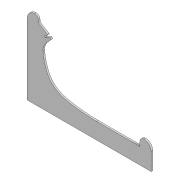
# Autodesk Inventor part: steep-rail
Saved by Autodesk Inventor 2020 (Build 240168000, 168)
## iProperties
Created: 2021-06-11
Part Number: steep-rail
Material: Generic
Document SubType Name: Modeling
Designer: Aidan Lee
Density: 1 g/cm^3
Appearance: Default
Author: Aidan Lee
Autodesk Inventor part; units mm, degrees
ref_plane "YZ Plane" through (0, 0, 0) normal (1, 0, 0) x (0, 1, 0)
ref_plane "XZ Plane" through (0, 0, 0) normal (0, 1, 0) x (-1, 0, 0)
ref_plane "XY Plane" through (0, 0, 0) normal (0, 0, 1) x (1, 0, 0)
sketch "Sketch3" plane through (0, 0, 0) normal (0, 0, 1) x (1, 0, 0)
  circle A0 centre (368.0481, 50) radius 50 construction
  line L0 (368.0481, 0) -> (514.9541, 0) construction
  line L1 (368.0481, 50) -> (514.9541, 50) construction
  line L2 (368.0481, 100) -> (514.9541, 100) construction
  line L3 (368.0481, 50) -> (343.0481, 6.6987) construction
  line L4 (368.0481, 50) -> (324.7469, 25) construction
  line L5 (368.0481, 50) -> (324.7469, 75) construction
  line L6 (343.0481, 93.3013) -> (368.0481, 50) construction
  line L7 (393.0481, 93.3013) -> (368.0481, 50) construction
  line L8 (411.3494, 75) -> (368.0481, 50) construction
  line L9 (411.3494, 25) -> (368.0481, 50) construction
  line L10 (393.0481, 6.6987) -> (368.0481, 50) construction
  line L11 (368.0481, 0) -> (368.0481, 100) construction
  line L12 (418.0481, 50) -> (368.0481, 50) construction
  line L13 (341.8682, 0) -> (341.8682, 100) construction
  line L14 (315.6883, 0) -> (315.6883, 100) construction
  line L15 (289.5083, 0) -> (289.5083, 100) construction
  line L16 (263.3284, 0) -> (263.3284, 100) construction
  line L17 (237.1485, 0) -> (237.1485, 100) construction
  line L18 (210.9685, 0) -> (210.9685, 100) construction
  line L19 (184.7886, 0) -> (184.7886, 100) construction
  line L20 (158.6086, 0) -> (158.6086, 100) construction
  circle A1 centre (315.6883, 50) radius 50 construction
  circle A2 centre (341.8682, 50) radius 50 construction
  circle A3 centre (289.5083, 50) radius 50 construction
  circle A4 centre (263.3284, 50) radius 50 construction
  circle A5 centre (237.1485, 50) radius 50 construction
  circle A6 centre (210.9685, 50) radius 50 construction
  line L21 (393.0481, 6.6987) -> (514.9541, 6.6987) construction
  line L22 (411.3494, 25) -> (514.9541, 25) construction
  line L23 (411.3494, 75) -> (514.9541, 75) construction
  line L24 (411.3494, 75) -> (514.9541, 75) construction
  line L25 (393.0481, 93.3013) -> (514.9541, 93.3013) construction
  line L26 (358.9895, 75) -> (339.5083, 50) construction
  line L27 (339.5083, 50) -> (306.6297, 25) construction
  line L28 (306.6297, 25) -> (262.1485, 6.6987) construction
  line L29 (262.1485, 6.6987) -> (210.9685, 0) construction
  line L30 (105.4843, -12.0642) -> (105.4843, 125.3083) construction
  line L31 (25.75, 0) -> (25.75, 23)
  line L32 (45.75, 17) -> (45.75, -21.2379)
  arc A7 (32.75, 30) -> (25.75, 23) centre (32.75, 23) ccw
  arc A8 (45.75, 17) -> (32.75, 30) centre (32.75, 17) ccw
  line L33 (32.75, 17) -> (45.75, 17) construction
  line L34 (32.75, 17) -> (32.75, 30) construction
  arc A9 (0, 0) -> (8.875, -12.2379) centre (12.875, 0) ccw
  arc A10 (16.875, -12.2379) -> (25.75, 0) centre (12.875, 0) ccw
  line L35 (45.75, -21.2379) -> (16.875, -21.2379)
  line L36 (8.875, -21.2379) -> (-177.0796, -21.2379)
  circle A11 centre (-144.2046, 110.3653) radius 12.875 construction
  line L37 (8.875, -21.2379) -> (8.875, -12.2379)
  line L38 (16.875, -21.2379) -> (16.875, -12.2379)
  line L39 (411.3494, 75) -> (158.6086, 75) construction
  line L40 (368.0481, 100) -> (158.6086, 100) construction
  line L41 (418.0481, 50) -> (158.6086, 50) construction
  line L42 (411.3494, 25) -> (158.6086, 25) construction
  line L43 (393.0481, 6.6987) -> (158.6086, 6.6987) construction
  line L44 (393.0481, 93.3013) -> (158.6086, 93.3013) construction
  line L45 (358.9895, 75) -> (366.8682, 93.3013) construction
  line L46 (366.8682, 93.3013) -> (368.0481, 100) construction
  spline S0 degree 4 poles (-157.0796, 100) (-157.0796, 88.9946) (-147.011, 72.6811) (-131.8577, 48.7932) (-88.4777, 17.6268) (-50.0176, 3.937) (-18.8717, 0) (0, 0) knots 0 0 0 0 0 0.264547 0.457223 0.66608 1 1 1 1 1
  line L47 (-157.0796, 100) -> (-157.0796, 81.2146) construction
  line L48 (0, 0) -> (-42.8818, 0) construction
  line L49 (-157.0796, 100) -> (-157.0796, 113)
  line L50 (-144.2046, 110.3653) -> (-157.0796, 110.3653) construction
  line L51 (-147.6984, 94.0277) -> (-120.1158, 108.3975) construction
  line L52 (-157.0796, 100) -> (0, 0) construction
  circle A12 centre (-147.2046, 105.4197) radius 9.875 construction
  line L53 (-147.2046, 105.4197) -> (-157.0796, 105.4197) construction
  line L54 (-146.1623, 94.828) -> (-144.7762, 92.1674) construction
  line L55 (-144.7762, 92.1674) -> (-142.2689, 93.4736) construction
  line L56 (-177.0796, 107) -> (-177.0796, -21.2379)
  arc A13 (-157.0796, 113) -> (-164.0796, 120) centre (-164.0796, 113) ccw
  line L57 (-164.0796, 113) -> (-164.0796, 120) construction
  line L58 (-164.0796, 113) -> (-157.0796, 113) construction
  arc A14 (-164.0796, 120) -> (-177.0796, 107) centre (-164.0796, 107) ccw
  line L59 (-164.0796, 107) -> (-177.0796, 107) construction
  line L60 (-164.0796, 107) -> (-164.0796, 120) construction
  line L61 (-457.0796, 100) -> (-300, 0)
  line L62 (-757.0796, 100) -> (-757.0796, 76.4376)
  line L63 (-600, 0) -> (-652.3765, 0)
  spline S1 degree 4 poles (-757.0796, 76.4376) (-757.0796, 65.0585) (-753.7776, 47.1407) (-745.4013, 7.8331) (-693.0053, 2.4317) (-668.8587, 0) (-652.3765, 0) knots 0 0 0 0 0 0.348765 0.598765 1 1 1 1 1
  line L64 (-477.0796, 107) -> (-477.0796, -21.2379)
  arc A15 (-464.0796, 120) -> (-477.0796, 107) centre (-464.0796, 107) ccw
  arc A16 (-457.0796, 113) -> (-464.0796, 120) centre (-464.0796, 113) ccw
  line L65 (-457.0796, 100) -> (-457.0796, 113)
  circle A17 centre (-447.2046, 105.4197) radius 9.875 construction
  circle A18 centre (-444.2046, 110.3653) radius 12.875 construction
  line L66 (-457.0796, 100) -> (-300, 0) construction
  line L67 (-447.6984, 94.0277) -> (-420.1158, 108.3975) construction
  line L68 (-444.7762, 92.1674) -> (-442.2689, 93.4736) construction
  line L69 (-446.1623, 94.828) -> (-444.7762, 92.1674) construction
  line L70 (-291.125, -21.2379) -> (-477.0796, -21.2379)
  arc A19 (-300, 0) -> (-291.125, -12.2379) centre (-287.125, 0) ccw
  line L71 (-291.125, -21.2379) -> (-291.125, -12.2379)
  line L72 (-283.125, -21.2379) -> (-283.125, -12.2379)
  arc A20 (-283.125, -12.2379) -> (-274.25, 0) centre (-287.125, 0) ccw
  line L73 (-254.25, -21.2379) -> (-283.125, -21.2379)
  line L74 (-254.25, 17) -> (-254.25, -21.2379)
  line L75 (-274.25, 0) -> (-274.25, 23)
  arc A21 (-267.25, 30) -> (-274.25, 23) centre (-267.25, 23) ccw
  arc A22 (-254.25, 17) -> (-267.25, 30) centre (-267.25, 17) ccw
  line L76 (-777.0796, 107) -> (-777.0796, -21.2379)
  arc A23 (-764.0796, 120) -> (-777.0796, 107) centre (-764.0796, 107) ccw
  arc A24 (-757.0796, 113) -> (-764.0796, 120) centre (-764.0796, 113) ccw
  line L77 (-757.0796, 100) -> (-757.0796, 113)
  circle A25 centre (-747.2046, 105.4197) radius 9.875 construction
  circle A26 centre (-744.2046, 110.3653) radius 12.875 construction
  line L78 (-757.0796, 100) -> (-600, 0) construction
  line L79 (-747.6984, 94.0277) -> (-720.1158, 108.3975) construction
  line L80 (-744.7762, 92.1674) -> (-742.2689, 93.4736) construction
  line L81 (-746.1623, 94.828) -> (-744.7762, 92.1674) construction
  line L82 (-591.125, -21.2379) -> (-777.0796, -21.2379)
  arc A27 (-600, 0) -> (-591.125, -12.2379) centre (-587.125, 0) ccw
  line L83 (-591.125, -21.2379) -> (-591.125, -12.2379)
  line L84 (-583.125, -21.2379) -> (-583.125, -12.2379)
  arc A28 (-583.125, -12.2379) -> (-574.25, 0) centre (-587.125, 0) ccw
  line L85 (-554.25, -21.2379) -> (-583.125, -21.2379)
  line L86 (-554.25, 17) -> (-554.25, -21.2379)
  line L87 (-574.25, 0) -> (-574.25, 23)
  arc A29 (-567.25, 30) -> (-574.25, 23) centre (-567.25, 23) ccw
  arc A30 (-554.25, 17) -> (-567.25, 30) centre (-567.25, 17) ccw
  line L88 (32.75, -233) -> (45.75, -233) construction
  line L89 (32.75, -233) -> (32.75, -220) construction
  arc A31 (45.75, -233) -> (32.75, -220) centre (32.75, -233) ccw construction
  line L90 (25.75, -250) -> (25.75, -227) construction
  line L91 (45.75, -233) -> (45.75, -271.2379) construction
  arc A32 (16.875, -262.2379) -> (25.75, -250) centre (12.875, -250) ccw construction
  line L92 (45.75, -271.2379) -> (16.875, -271.2379) construction
  arc A33 (0, -250) -> (8.875, -262.2379) centre (12.875, -250) ccw construction
  arc A34 (32.75, -220) -> (25.75, -227) centre (32.75, -227) ccw construction
  line L93 (8.875, -271.2379) -> (-177.0796, -271.2379) construction
  line L94 (-157.0796, -150) -> (0, -250) construction
  spline S2 degree 4 poles (-157.0796, -150) (-157.0796, -161.0054) (-147.011, -177.3189) (-131.8577, -201.2068) (-88.4777, -232.3732) (-50.0176, -246.063) (-18.8717, -250) (0, -250) knots 0 0 0 0 0 0.264547 0.457223 0.66608 1 1 1 1 1 construction
  line L95 (-177.0796, -143) -> (-177.0796, -271.2379)
  line L96 (-146.1623, -155.172) -> (-144.7762, -157.8326) construction
  line L97 (-144.7762, -157.8326) -> (-142.2689, -156.5264) construction
  line L98 (-147.6984, -155.9723) -> (-120.1158, -141.6025) construction
  line L99 (-157.0796, -150) -> (-157.0796, -168.7854) construction
  line L100 (-147.2046, -144.5803) -> (-157.0796, -144.5803) construction
  line L101 (-144.2046, -139.6347) -> (-157.0796, -139.6347) construction
  circle A35 centre (-147.2046, -144.5803) radius 9.875 construction
  line L102 (0, -250) -> (-42.8818, -250) construction
  line L103 (16.875, -271.2379) -> (16.875, -262.2379) construction
  line L104 (8.875, -271.2379) -> (8.875, -262.2379) construction
  circle A36 centre (-144.2046, -139.6347) radius 12.875 construction
  line L105 (-164.0796, -143) -> (-177.0796, -143) construction
  line L106 (-157.0796, -150) -> (-157.0796, -137) construction
  line L107 (-164.0796, -137) -> (-157.0796, -137) construction
  arc A37 (-157.0796, -137) -> (-164.0796, -130) centre (-164.0796, -137) ccw
  line L108 (-164.0796, -137) -> (-164.0796, -130) construction
  line L109 (-164.0796, -143) -> (-164.0796, -130) construction
  arc A38 (-164.0796, -130) -> (-177.0796, -143) centre (-164.0796, -143) ccw
  arc A39 (32.75, -227) -> (25.75, -234) centre (32.75, -234) ccw
  line L110 (32.75, -234) -> (25.75, -234) construction
  line L111 (32.75, -234) -> (32.75, -227) construction
  line L112 (45.75, -271.2379) -> (-177.0796, -271.2379)
  arc A40 (45.75, -240) -> (32.75, -227) centre (32.75, -240) ccw
  line L113 (32.75, -240) -> (45.75, -240) construction
  line L114 (32.75, -240) -> (32.75, -227) construction
  line L115 (45.75, -240) -> (45.75, -271.2379)
  line L116 (0, -242) -> (25.75, -242)
  line L117 (25.75, -234) -> (25.75, -242)
  line L118 (-149.0796, -145.6094) -> (-149.0796, -150)
  line L119 (-149.0796, -145.6094) -> (-157.0796, -140.5164)
  line L120 (-157.0796, -140.5164) -> (-157.0796, -137)
  line L121 (57.9242, -250) -> (-50.1018, -250) construction
  spline S3 degree 4 poles (-149.0796, -150) (-149.0796, -154.1011) (-147.2668, -159.7716) (-135.8793, -178.0796) (-120.229, -197.0865) (-83.3361, -225.9308) (-47.2959, -235.9761) (-18.0598, -242) (0, -242) knots 0 0 0 0 0 0.173174 0.31592 0.488873 0.682943 1 1 1 1 1
  line L122 (-158.9844, -148.7874) -> (-160.5796, -147.7718) construction
  line L123 (-149.0796, -145.6094) -> (2.3304, -242) construction
  line L124 (-149.0796, -145.6094) -> (-139.5059, -151.7042)
  line L125 (-146.1623, -155.172) -> (-139.5059, -151.7042)
  line L126 (-144.7762, -157.8326) -> (-146.1623, -155.172)
  line L127 (-144.7762, -157.8326) -> (-136.5837, -153.5646)
  line L128 (-136.5837, -153.5646) -> (-134.053, -155.1756)
  line L129 (-136.5837, -153.5646) -> (-136.7042, -153.7538) construction
  line L130 (-134.053, -155.1756) -> (-134.1481, -155.3251) construction
  spline S4 degree 4 poles (-134.053, -155.1756) (-136.3893, -157.4676) (-136.0613, -162.1246) (-140.7447, -169.8773) (-137.1035, -175.12) knots 0 0 0 0 0 1 1 1 1 1
  line L131 (-134.053, -155.1756) -> (-131.4385, -154.0999) construction
  line L132 (-254.25, -271.2379) -> (-477.0796, -271.2379)
  line L133 (-477.0796, -143) -> (-477.0796, -271.2379)
  arc A41 (-464.0796, -130) -> (-477.0796, -143) centre (-464.0796, -143) ccw
  arc A42 (-457.0796, -137) -> (-464.0796, -130) centre (-464.0796, -137) ccw
  line L134 (-457.0796, -140.5164) -> (-457.0796, -137)
  line L135 (-449.0796, -145.6094) -> (-457.0796, -140.5164)
  line L136 (-449.0796, -145.6094) -> (-439.5059, -151.7042)
  line L137 (-446.1623, -155.172) -> (-439.5059, -151.7042)
  line L138 (-444.7762, -157.8326) -> (-446.1623, -155.172)
  line L139 (-444.7762, -157.8326) -> (-436.5837, -153.5646)
  line L140 (-436.5837, -153.5646) -> (-434.053, -155.1756)
  line L141 (-449.0796, -145.6094) -> (-297.6696, -242) construction
  line L142 (-300, -242) -> (-274.25, -242)
  line L143 (-274.25, -234) -> (-274.25, -242)
  arc A43 (-267.25, -227) -> (-274.25, -234) centre (-267.25, -234) ccw
  arc A44 (-254.25, -240) -> (-267.25, -227) centre (-267.25, -240) ccw
  line L144 (-254.25, -240) -> (-254.25, -271.2379)
  circle A45 centre (-447.2046, -144.5803) radius 9.875 construction
  line L145 (-457.0796, -150) -> (-300, -250) construction
  circle A46 centre (-444.2046, -139.6347) radius 12.875 construction
  line L146 (-554.25, -271.2379) -> (-777.0796, -271.2379)
  line L147 (-777.0796, -143) -> (-777.0796, -271.2379)
  arc A47 (-764.0796, -130) -> (-777.0796, -143) centre (-764.0796, -143) ccw
  arc A48 (-757.0796, -137) -> (-764.0796, -130) centre (-764.0796, -137) ccw
  line L148 (-757.0796, -140.5164) -> (-757.0796, -137)
  line L149 (-749.0796, -145.6094) -> (-757.0796, -140.5164)
  line L150 (-749.0796, -145.6094) -> (-739.5059, -151.7042)
  line L151 (-746.1623, -155.172) -> (-739.5059, -151.7042)
  line L152 (-744.7762, -157.8326) -> (-746.1623, -155.172)
  line L153 (-744.7762, -157.8326) -> (-736.5837, -153.5646)
  line L154 (-736.5837, -153.5646) -> (-734.053, -155.1756)
  line L155 (-749.0796, -145.6094) -> (-597.6696, -242) construction
  line L156 (-600, -242) -> (-574.25, -242)
  line L157 (-574.25, -234) -> (-574.25, -242)
  arc A49 (-567.25, -227) -> (-574.25, -234) centre (-567.25, -234) ccw
  arc A50 (-554.25, -240) -> (-567.25, -227) centre (-567.25, -240) ccw
  line L158 (-554.25, -240) -> (-554.25, -271.2379)
  circle A51 centre (-747.2046, -144.5803) radius 9.875 construction
  line L159 (-757.0796, -150) -> (-600, -250) construction
  circle A52 centre (-744.2046, -139.6347) radius 12.875 construction
  line L160 (-297.6696, -242) -> (-434.053, -155.1756)
  spline S5 degree 4 poles (-757.0796, -173.5624) (-757.0796, -184.9415) (-753.7776, -202.8593) (-745.4013, -242.1669) (-693.0053, -247.5683) (-668.8587, -250) (-652.3765, -250) knots 0 0 0 0 0 0.348765 0.598765 1 1 1 1 1 construction
  line L161 (-757.0796, -150) -> (-757.0796, -173.5624)
  line L162 (-600, -250) -> (-652.3765, -250) construction
  line L163 (-600, -242) -> (-652.3765, -242)
  spline S6 degree 4 poles (-749.0796, -173.5624) (-749.0796, -183.7991) (-746.0176, -199.7502) (-737.9559, -236.335) (-690.8375, -239.2991) (-667.8077, -242) (-652.3765, -242) knots 0 0 0 0 0 0.346383 0.596383 1 1 1 1 1
  line L164 (-749.0796, -173.5624) -> (-749.0796, -170.035) construction
  spline S7 degree 3 poles (-734.053, -155.1756) (-737.3254, -159.7583) (-749.7015, -168.859) (-748.818, -180.0805) knots 0 0 0 0 1 1 1 1
  point P0 (158.6086, 0)
  point P1 (-148.021, 75)
  point P2 (-128.5398, 50)
  point P3 (-95.6611, 25)
  point P4 (-51.1799, 6.6987)
  point P5 (-155.8997, 93.3013)
  point P6 (-753.2027, 48.1984)
  point P7 (-737.7866, 19.9116)
  point P8 (-697.6619, 3.8098)
  point P9 (-457.0796, 110.3653)
  point P10 (-457.0796, 105.4197)
  point P11 (-757.0796, 110.3653)
  point P12 (-757.0796, 105.4197)
  point P13 (-51.1799, -243.3013)
  point P14 (-95.6611, -225)
  point P15 (-148.021, -175)
  point P16 (-128.5398, -200)
  point P17 (-155.8997, -156.6987)
  point P18 (-157.0796, -141.4334)
  point P19 (-153.0796, -143.0629)
  point P20 (-152.1421, -144.5803)
  point P21 (3.9112, -250)
  point P22 (-147.2046, -158.2164)
  point P23 (-137.7547, -174.1759)
  point P24 (-121.904, -193.5196)
  point P25 (-91.5665, -216.9339)
  point P26 (-48.8291, -234.4712)
  point P27 (-135.7448, -158.2544)
  point P28 (-137.814, -165.5952)
  point P29 (-453.0796, -143.0629)
  point P30 (-457.0796, -144.5803)
  point P31 (-447.6984, -155.9723)
  point P32 (-457.0796, -139.6347)
  point P33 (-753.0796, -143.0629)
  point P34 (-757.0796, -144.5803)
  point P35 (-747.6984, -155.9723)
  point P36 (-757.0796, -139.6347)
  point P37 (-753.2027, -201.8016)
  point P38 (-737.7866, -230.0884)
  point P39 (-697.6619, -246.1902)
  point P40 (-745.4939, -198.9007)
  point P41 (-731.3987, -224.5882)
  point P42 (-695.3384, -238.4632)
  point P43 (-741.9622, -163.8871)
  point P44 (-300, 0)
  dimension "d43" = 25.75
  dimension "d53" = 19.75
  dimension "diameter" = 100
  dimension "d8" = 26.1799
  dimension "d14" = 30
  dimension "d15" = 30
  dimension "d16" = 30
  dimension "d26" = 90
  dimension "stopper" = 30
  dimension "stopperthickness" = 20
  dimension "d32" = 12.875
  dimension "d33" = 12.875
  dimension "d38" = 6
  dimension "d47" = 8
  dimension "d49" = 9
  dimension "d55" = 120
  dimension "d56" = 3
  dimension "d57" = 90
  dimension "d58" = 90
  dimension "d59" = 20
  dimension "d60" = 6
  dimension "d61" = 20
  dimension "d62" = 28.875
  dimension "d72" = 300
  dimension "d93" = 250
  dimension "d98" = 90
  dimension "d99" = 44.2379
  dimension "d100" = 37.2379
  dimension "d101" = 90
  dimension "railheight" = 8
  dimension "d104" = 8
  dimension "d105" = 8
  dimension "d106" = 3
  dimension "d109" = 300
  dimension "d116" = 250
  dimension "d121" = 8
  constraints: 328 end point, 78 point on circle, 46 point on line, 39 centre point, 35 horizontal, 24 horizontal alignment, 24 vertical, 12 perpendicular, 11 vertical alignment, 10 midpoint, 8 coincident, 7 symmetric about line, 4 collinear, 3 parallel, 2 equal length, 2 tangent, 377 other
  measures "d8" distance of L11.start L13.start
  measures "d14" angle of L6 L11
  measures "d15" angle of L11 L7
  measures "d16" angle of L9 L12
  measures "d26" angle of L33 L34
  measures "stopper" vertical distance of L34.end A9.centre
  measures "stopperthickness" distance between parallel lines of L31 L32
  measures "d32" radius of A9
  measures "d33" radius of A10
  measures "d38" vertical distance of L32.start L31.end
  measures "d47" distance between parallel lines of L37 L38
  measures "d49" distance of L36.start L37.end
  measures "d55" angle of L52 L51
  measures "d56" distance between parallel lines of L55 L51
  measures "d57" angle of L58 L57
  measures "d58" angle of L60 L59
  measures "d59" distance between parallel lines of L56 L49
  measures "d60" distance of L59.start L57.start
  measures "d61" vertical distance of L57.end L47.start
  measures "d62" distance between parallel lines of L32 L38
  measures "d72" distance of L56.start L64.start
  measures "d93" distance of L32.start L88.end
  measures "d98" angle of L111 L110
  measures "d99" distance from line of L35 A7.centre
  measures "d100" distance from line of L112 L110.start
  measures "d101" angle of L113 L114
  measures "railheight" distance from line of L106.end L118
  measures "d104" distance between parallel lines of L116 L121
  measures "d105" distance between parallel lines of L122 L119
  measures "d106" distance between parallel lines of L130 L129
  measures "d109" distance of L91.end L132.start
  measures "d116" distance of L62.end L161.end
  measures "d121" distance between parallel lines of L161 L164
extrude "Extrusion1" add sketch "Sketch3" along normal blind 3 contours L146 L147 A47 A48 L148 L149 L150 L151 L152 L153 L154 S7 S6 L163 L156 L157 A49 A50 L158
fillet "Fillet2" radius 1 1 edges at (-739.5059, -151.7042, 1.5)
equation "\"d8\" = 0.261799 * diameter"
body "Solid1"
